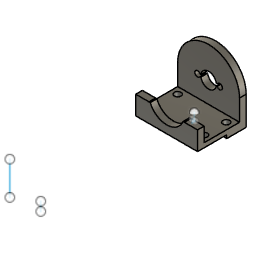
モーター土台03 v2 (Autodesk Fusion 360 design; units mm, degrees)
Autodesk Fusion 360 part; units mm, degrees
sketch "スケッチ1" plane through (0, 0, 0) normal (0, 0, 1) x (1, 0, 0)
  line L0 (0, 0) -> (-28, 0)
  line L1 (-28, 0) -> (-28, -22)
  line L2 (-28, -22) -> (0, -22)
  line L3 (0, -22) -> (0, 0)
  line L4 (0, 0) -> (0, -6)
  line L5 (0, -6) -> (-3, -6)
  line L6 (0, -22) -> (0, -16)
  line L7 (0, -16) -> (-3, -16)
  line L8 (-28, -22) -> (-28, -16)
  line L9 (-28, -16) -> (-25, -16)
  line L10 (-28, 0) -> (-28, -6)
  line L11 (-28, -6) -> (-25, -6)
  circle A0 centre (-25, -6) radius 1.5
  circle A1 centre (-25, -16) radius 1.5
  circle A2 centre (-3, -6) radius 1.5
  circle A3 centre (-3, -16) radius 1.5
  dimension "d1" = 28
  dimension "d2" = 22
  constraint horizontal L0
  constraint vertical L1
  constraint horizontal L2
  constraint vertical L3
  constraint coincident L0.start L3.end
  constraint coincident L3 L4.end
  constraint perpendicular L0 L4
  constraint perpendicular L3 L5
  constraint coincident L3 L6.end
  constraint perpendicular L6 L7
  constraint coincident L1 L8.end
  constraint perpendicular L8 L9
  constraint coincident L1 L10.end
  constraint perpendicular L10 L11
  constraint coincident L11.end A0.centre
  constraint coincident L9.end A1.centre
  constraint coincident L5.end A2.centre
  constraint coincident L7.end A3.centre
  measures "d1" distance of L0.start L0.end
  measures "d2" distance of L0.start L2.end
extrude "押し出し1" add sketch "スケッチ1" along normal blind 2
sketch "スケッチ2" plane through (0, 0, 0) normal (0, 1, 0) x (1, 0, 0)
  line L0 (0, -2) -> (0, -13)
  line L1 (-28, -2) -> (-28, -13)
  line L2 (-17.8, -15.5) -> (-18.134, -15.5)
  line L3 (-17.8, -15.5) -> (-17.4641, -15.5)
  line L4 (-17.8, -14.5) -> (-17.4641, -14.5)
  line L5 (-17.8, -14.5) -> (-18.134, -14.5)
  line L6 (-10.5, -15.5) -> (-10.5359, -15.5)
  line L7 (-10.5, -15.5) -> (-9.866, -15.5)
  line L8 (-10.3, -14.5) -> (-10.5359, -14.5)
  line L9 (-10.3, -14.5) -> (-9.866, -14.5)
  arc A0 (-17.4641, -15.5) -> (-10.5352, -15.495) centre (-14, -15) ccw
  arc A1 (-10.5359, -14.5) -> (-17.4641, -14.5) centre (-14, -15) ccw
  arc A2 (-9.866, -15.5) -> (-9.866, -14.5) centre (-9, -15) ccw
  arc A3 (-18.134, -14.5) -> (-18.134, -15.5) centre (-19, -15) ccw
  line L10 (-28, -13) -> (-28, -15)
  line L11 (0, -13) -> (0, -15)
  arc A4 (-28, -15) -> (0, -15) centre (-14, -15) ccw
  line L12 (-28, -2) -> (0, -2)
  constraint vertical L0
  constraint horizontal L2
  constraint parallel L2 L3
  constraint parallel L3 L4
  constraint parallel L4 L5
  constraint parallel L4 L6
  constraint parallel L6 L7
  constraint horizontal L8
  constraint parallel L8 L9
  constraint coincident A0.centre A1.centre
  constraint parallel L1 L10
  constraint vertical L11
  constraint perpendicular L0 L12
extrude "押し出し2" add sketch "スケッチ2" against normal blind 3
sketch "スケッチ3" plane through (0, 0, 0) normal (0, 1, 0) x (1, 0, 0)
sketch "スケッチ4" plane through (0, 0, 0) normal (1, 0, 0) x (0, 1, 0)
move_body "移動1" bodies 1 to x (1, 0, 0) y (0, 1, 0) z (0, 0, 1) at (0, 22, 0)
sketch "スケッチ5" plane through (0, 0, 0) normal (0, 1, 0) x (1, 0, 0)
  line L0 (0, -2) -> (0, -12)
  line L1 (-28, -2) -> (-28, -12)
  line L2 (-28, -12) -> (-22, -12)
  line L3 (0, -12) -> (-6, -12)
  arc A0 (-6, -12) -> (-22, -12) centre (-14, -15) ccw
  line L4 (-28, -2) -> (0, -2)
  constraint vertical L0
  constraint vertical L1
  constraint perpendicular L1 L2
  constraint perpendicular L0 L3
  constraint perpendicular L0 L4
extrude "押し出し3" add sketch "スケッチ5" along normal blind 3
sketch "スケッチ6" plane through (0, 0, 0) normal (0, 0, 1) x (1, 0, 0)
sketch "スケッチ7" plane through (0, 0, 0) normal (0, 1, 0) x (1, 0, 0)
sketch "スケッチ8" plane through (0, 0, 0) normal (0, 0, 1) x (1, 0, 0)
move_body "移動2" bodies 1 to x (1, 0, 0) y (0, 1, 0) z (0, 0, 1) at (0, -22, 0)
sketch "スケッチ9" plane through (0, 0, 0) normal (0, 1, 0) x (1, 0, 0)
  circle A0 centre (-19, -15) radius 1.25
  circle A1 centre (-9, -15) radius 1.25
  dimension "d9" = 2.5
  dimension "d10" = 2.5
  measures "d9" diameter of A0
  measures "d10" diameter of A1
extrude "押し出し4" cut sketch "スケッチ9" against normal blind 3
sketch "スケッチ10" plane through (0, 0, 0) normal (1, 0, 0) x (0, 1, 0)
sketch "スケッチ11" plane through (0, 0, 0) normal (0, 0, 1) x (1, 0, 0)
sketch "スケッチ12" plane through (0, 0, 0) normal (1, 0, 0) x (0, 1, 0)
sketch "スケッチ13" plane through (0, 0, 0) normal (0, 1, 0) x (1, 0, 0)
  line L0 (-14, -15) -> (-14, 0)
  constraint vertical L0
sketch "スケッチ14" plane through (0, 0, 0) normal (0, 0, 1) x (1, 0, 0)
move_body "移動3" bodies 1 to x (1, 0, 0) y (0, 1, 0) z (0, 0, 1) at (14, 0, 0)
move_body "移動4" bodies 1 to x (1, 0, 0) y (0, 1, 0) z (0, 0, 1) at (0, 79, 0)
sketch "スケッチ15" plane through (0, 0, 0) normal (0, 0, 1) x (1, 0, 0)
  circle A0 centre (0, 0) radius 70
  dimension "d13" = 140
  constraint coincident A0.centre origin
  measures "d13" diameter of A0
sketch "スケッチ16" plane through (0, 0, 0) normal (1, 0, 0) x (0, 1, 0)
extrude "押し出し5" cut sketch "スケッチ15" along normal blind 1.5
extrude "押し出し6" add 1 faces at (3.2162, 66.5503, 2) along direction (0, 0, 1) blind 0.5
sketch "スケッチ17" plane through (0, 0, 0) normal (1, 0, 0) x (0, 1, 0)
sketch "スケッチ18" plane through (0, 0, 0) normal (0, 1, 0) x (1, 0, 0)
  line L0 (0, -1.5) -> (0, -5.5)
  constraint vertical L0
extrude "押し出し7" add 1 faces at (3.2162, 66.5503, 2.5) along direction (0, 0, 1) blind 3
sketch "スケッチ19" plane through (0, 0, 0) normal (1, 0, 0) x (0, 1, 0)
extrude "押し出し8" cut 1 faces at (-1.5649, 65.1318, 1.5) along direction (0, 0, 1) blind 2
sketch "スケッチ20" plane through (0, 0, 0) normal (1, 0, 0) x (0, 1, 0)
  line L0 (69.5, 5.5) -> (69.5, 2.5)
  line L1 (68.6, 3.5) -> (68.6, 2)
  line L2 (68.6, 2) -> (69.9, 2)
  line L3 (69.5, 2.5) -> (69.5, 2)
  constraint vertical L0
  constraint parallel L0 L1
  constraint perpendicular L1 L2
  constraint coincident L2 L3.end
  constraint perpendicular L2 L3
extrude "押し出し9" cut 1 faces at (3.3549, 77.3909, 0) along direction (0, 0, 1) blind 2
sketch "スケッチ21" plane through (0, 0, 0) normal (1, 0, 0) x (0, 1, 0)
sketch "スケッチ22" plane through (0, 0, 0) normal (0, 0, 1) x (1, 0, 0)
sketch "スケッチ23" plane through (0, 0, 0) normal (0, 0, 1) x (1, 0, 0)
  circle A0 centre (0, 0) radius 71.5
  dimension "d24" = 143
  constraint coincident A0.centre origin
  measures "d24" diameter of A0
extrude "押し出し10" cut sketch "スケッチ23" along normal blind 3.5
extrude "押し出し11" add 1 faces at (1.5645, 76.4486, 2) along direction (0, 0, -1) blind 2
sketch "スケッチ24" plane through (0, 0, 0) normal (0, 1, 0) x (1, 0, 0)
  arc A0 (8, -12) -> (-8, -12) centre (0, -15) ccw
  line L0 (-8, -12) -> (8, -12)
extrude "押し出し12" add sketch "スケッチ24" along normal blind 60
sketch "スケッチ25" plane through (0, 0, 0) normal (0, 1, 0) x (1, 0, 0)
  line L0 (14, -12) -> (-14, -12)
  arc A0 (7.4162, -12) -> (-7.4162, -12) centre (0, -15) ccw
  dimension "d31" = 8
  constraint horizontal L0
  constraint coincident L0 A0.end
  constraint coincident L0 A0.start
  measures "d31" radius of A0
extrude "押し出し13" cut sketch "スケッチ25" along normal blind 60
extrude "押し出し14" cut 1 faces at (-0.5969, 0, 6.8552) along direction (0, 1, 0) blind 57
sketch "スケッチ26" plane through (0, 0, 0) normal (1, 0, 0) x (0, 1, 0)
extrude "押し出し15" cut 1 faces at (1.5645, 76.4486, 0) along direction (0, 0, 1) blind 2
